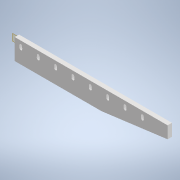
# Autodesk Inventor part: guide rails
Saved by Autodesk Inventor 2020 (Build 240168000, 168)
## iProperties
Created: 2020-02-12
Part Number: guide rails
Material: Generic
Document SubType Name: Modeling
Designer: jackm
Density: 1 g/cm^3
Appearance: Default
Author: jackm
Autodesk Inventor part; units mm, degrees
ref_plane "YZ Plane" through (0, 0, 0) normal (1, 0, 0) x (0, 1, 0)
ref_plane "XZ Plane" through (0, 0, 0) normal (0, 1, 0) x (-1, 0, 0)
ref_plane "XY Plane" through (0, 0, 0) normal (0, 0, 1) x (1, 0, 0)
ref_plane "Work Plane1" through (0, 0, 0) normal (0, 0, 1) x (1, 0, 0)
sketch "Sketch1" plane through (0, 0, 0) normal (0, 0, 1) x (1, 0, 0)
  circle A0 centre (59.69, -4.445) radius 1.9304 construction
  circle A1 centre (161.29, -4.445) radius 1.9304 construction
  circle A2 centre (135.89, -4.445) radius 1.9304 construction
  circle A3 centre (34.29, -4.445) radius 1.9304 construction
  circle A4 centre (85.09, -4.445) radius 1.9304 construction
  circle A5 centre (186.69, -4.445) radius 1.9304 construction
  circle A6 centre (110.49, -4.445) radius 1.9304 construction
  circle A7 centre (8.89, -4.445) radius 1.9304 construction
  line L0 (0, 0) -> (0, -8.89) construction
  line L1 (0, -8.89) -> (195.58, -8.89) construction
  line L2 (195.58, 0) -> (195.58, -8.89) construction
  line L3 (0, 0) -> (195.58, 0) construction
  circle A8 centre (254.7602, -6.1683) radius 25.137 construction
  line L4 (0, 0) -> (0, -8.89)
  line L5 (0, -8.89) -> (0, -26.5684)
  line L6 (0, -26.5684) -> (127, -26.5684)
  line L7 (127, -26.5684) -> (223.5038, -13.8825)
  line L8 (223.5038, -13.8825) -> (223.5038, 0)
  line L9 (223.5038, 0) -> (223.5038, 3.81)
  line L10 (223.5038, 3.81) -> (0, 3.81)
  line L11 (0, 3.81) -> (0, 0)
  line L12 (188.7012, -6.3331) -> (188.62, -2.474)
  line L13 (184.6788, -6.3331) -> (184.76, -2.474)
  arc A9 (163.22, -2.474) -> (159.36, -2.474) centre (161.29, -2.5146) ccw
  arc A10 (159.2788, -6.3331) -> (163.3012, -6.3331) centre (161.29, -6.3754) ccw
  line L14 (163.3012, -6.3331) -> (163.22, -2.474)
  line L15 (159.2788, -6.3331) -> (159.36, -2.474)
  arc A11 (137.82, -2.474) -> (133.96, -2.474) centre (135.89, -2.5146) ccw
  line L16 (137.9012, -6.3331) -> (137.82, -2.474)
  line L17 (133.8788, -6.3331) -> (133.96, -2.474)
  arc A12 (108.4788, -6.3331) -> (112.5012, -6.3331) centre (110.49, -6.3754) ccw
  line L18 (112.5012, -6.3331) -> (112.42, -2.474)
  line L19 (108.4788, -6.3331) -> (108.56, -2.474)
  arc A13 (87.02, -2.474) -> (83.16, -2.474) centre (85.09, -2.5146) ccw
  arc A14 (83.0788, -6.3331) -> (87.1012, -6.3331) centre (85.09, -6.3754) ccw
  line L20 (87.1012, -6.3331) -> (87.02, -2.474)
  line L21 (83.0788, -6.3331) -> (83.16, -2.474)
  arc A15 (61.62, -2.474) -> (57.76, -2.474) centre (59.69, -2.5146) ccw
  arc A16 (57.6788, -6.3331) -> (61.7012, -6.3331) centre (59.69, -6.3754) ccw
  line L22 (61.7012, -6.3331) -> (61.62, -2.474)
  line L23 (57.6788, -6.3331) -> (57.76, -2.474)
  arc A17 (36.22, -2.474) -> (32.36, -2.474) centre (34.29, -2.5146) ccw
  arc A18 (32.2788, -6.3331) -> (36.3012, -6.3331) centre (34.29, -6.3754) ccw
  line L24 (36.3012, -6.3331) -> (36.22, -2.474)
  line L25 (32.2788, -6.3331) -> (32.36, -2.474)
  arc A19 (10.82, -2.474) -> (6.96, -2.474) centre (8.89, -2.5146) ccw
  arc A20 (6.8788, -6.3331) -> (10.9012, -6.3331) centre (8.89, -6.3754) ccw
  line L26 (10.9012, -6.3331) -> (10.82, -2.474)
  line L27 (6.8788, -6.3331) -> (6.96, -2.474)
  arc A21 (184.6788, -6.3331) -> (188.7012, -6.3331) centre (186.69, -6.3754) ccw
  arc A22 (188.62, -2.474) -> (184.76, -2.474) centre (186.69, -2.5146) ccw
  arc A23 (133.8788, -6.3331) -> (137.9012, -6.3331) centre (135.89, -6.3754) ccw
  arc A24 (112.42, -2.474) -> (108.56, -2.474) centre (110.49, -2.5146) ccw
  dimension "d0" = 17.6784
  dimension "d1" = 127
  dimension "d2" = 3.81
  constraints: 48 end point, 34 point on circle, 32 tangent, 16 centre point, 3 perpendicular, 1 parallel, 1 point on line, 1 vertical
  measures "d0" distance of L0.end L5.end
  measures "d1" distance of L5.end L6.end
  measures "d2" distance of L8.end L9.end
extrude "Extrusion1" add sketch "Sketch1" along normal blind 3.81
fillet "Fillet1" radius 127 1 edges at (127, -26.5684, 1.905)
body "Solid1"
